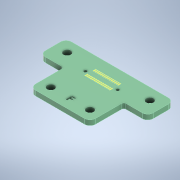
# Autodesk Inventor part: Out-facing Connector PCB
Saved by Autodesk Inventor 2021 (Build 250183000, 183)
## iProperties
Created: 2020-04-07
Part Number: Out-facing Connector PCB
Material: Phenolic Resin
Document SubType Name: Modeling
Designer: jgray
Density: 1.38 g/cm^3
Appearance: Smooth - Dark Sea Green
Author: jgray
Autodesk Inventor part; units mm, degrees
ref_plane "YZ Plane" through (0, 0, 0) normal (1, 0, 0) x (0, 1, 0)
ref_plane "XZ Plane" through (0, 0, 0) normal (0, 1, 0) x (-1, 0, 0)
ref_plane "XY Plane" through (0, 0, 0) normal (0, 0, 1) x (1, 0, 0)
sketch "Sketch1" plane through (0, 0, 0) normal (0, 1, 0) x (-1, 0, 0)
  line L0 (13.75, 0) -> (36.25, 0)
  line L1 (49.75, -18) -> (49.75, -25)
  line L2 (47.25, -27.5) -> (2.75, -27.5)
  line L3 (0.25, -25) -> (0.25, -18)
  line L4 (25, -34.1071) -> (25, 14.7902) construction
  line L5 (36.25, 0) -> (13.75, 0)
  line L6 (11.25, -2.5) -> (11.25, -14.5)
  line L7 (38.75, -14.5) -> (38.75, -2.5)
  line L8 (39.75, -15.5) -> (47.25, -15.5)
  line L9 (10.25, -15.5) -> (2.75, -15.5)
  arc A0 (38.75, -14.5) -> (39.75, -15.5) centre (39.75, -14.5) ccw
  arc A1 (10.25, -15.5) -> (11.25, -14.5) centre (10.25, -14.5) ccw
  arc A2 (49.75, -18) -> (47.25, -15.5) centre (47.25, -18) ccw
  arc A3 (47.25, -27.5) -> (49.75, -25) centre (47.25, -25) ccw
  arc A4 (2.75, -15.5) -> (0.25, -18) centre (2.75, -18) ccw
  arc A5 (0.25, -25) -> (2.75, -27.5) centre (2.75, -25) ccw
  arc A6 (38.75, -2.5) -> (36.25, 0) centre (36.25, -2.5) ccw
  arc A7 (13.75, 0) -> (11.25, -2.5) centre (13.75, -2.5) ccw
  point P0 (0, 0)
  point P1 (49.75, -27.5)
  point P2 (0.25, -27.5)
  point P3 (38.75, 0)
  point P4 (11.25, -1)
  point P5 (38.75, -1)
  point P6 (12.25, 0)
  dimension "d0" = 49.5
  dimension "d3" = 1
  dimension "d4" = 2.5
  dimension "d5" = 2.5
  dimension "d8" = 27.5
  dimension "d9" = 12
  dimension "d10" = 27.5
  dimension "d11" = 12
  dimension "d129" = 2.5
  dimension "d130" = 2.5
  constraints: 20 end point, 16 point on circle, 16 tangent, 10 point on line, 8 centre point, 3 equal radius, 3 parallel, 2 horizontal, 2 perpendicular, 1 vertical, 2 other
  measures "d0" distance of point (49.75, -27.5) point (0.25, -27.5)
  measures "d3" radius of A0
  measures "d4" radius of A2
  measures "d5" radius of A4
  measures "d8" distance between parallel lines of L2 L0
  measures "d9" distance between parallel lines of L2 L9
  measures "d10" distance between parallel lines of L7 L6
  measures "d11" distance between parallel lines of L2 L8
  measures "d129" radius of A6
  measures "d130" radius of A7
extrude "Extrusion1" add sketch "Sketch1" along normal blind 2.3
sketch "Sketch2" plane through (0, 2.3, 0) normal (0, 1, 0) x (1, 0, 0)
  line L0 (-48.4088, 22.25) -> (9.4819, 22.25) construction
  line L1 (-42.4458, 4.75) -> (-3.4379, 4.75) construction
  line L2 (-34, -3.7156) -> (-34, 9.7011) construction
  line L3 (-16, -3.7156) -> (-16, 9.7011) construction
  line L4 (-44, 10.4465) -> (-44, 20.1364) construction
  line L5 (-6, 8.2104) -> (-6, 20.1364) construction
  line L6 (-25, 27.2588) -> (-25, -6.0345) construction
  line L7 (-2.75, 27.5) -> (-47.25, 27.5) construction
  point P0 (0, 0)
  point P1 (-25, 27.5)
  point P2 (-44, 22.25)
  point P3 (-34, 4.75)
  point P4 (-16, 4.75)
  point P5 (-6, 22.25)
  dimension "d12" = 9
  dimension "d13" = 19
  dimension "d14" = 5.25
  dimension "d15" = 22.75
  constraints: 14 end point, 9 point on line, 4 vertical, 2 horizontal, 1 midpoint, 1 perpendicular, 2 other
  measures "d12" distance between parallel lines of L6 L3
  measures "d13" distance between parallel lines of L6 L4
  measures "d14" distance between parallel lines of L7 L0
  measures "d15" distance between parallel lines of L7 L1
hole "Hole1" at (-44, 2.3, -22.25) at (-34, 2.3, -4.75) at (-16, 2.3, -4.75) at (-6, 2.3, -22.25) direction (0, -1, 0) diameter 3.4 end through all clearance for "Countersunk Flat Head Screw ISO 2009/7046" size "M3" standard "ISO"
sketch "Sketch4" plane through (0, 2.3, 0) normal (0, 1, 0) x (1, 0, 0)
  circle A0 centre (-16, 4.75) radius 1.7 projected
  circle A1 centre (-44, 22.25) radius 1.7
  circle A2 centre (-34, 4.75) radius 1.7 projected
  circle A3 centre (-6, 22.25) radius 1.7 projected
  arc A4 (-10.25, 15.5) -> (-11.25, 14.5) centre (-10.25, 14.5) ccw projected
  line L0 (-10.25, 15.5) -> (-2.75, 15.5) projected
  arc A5 (-2.75, 15.5) -> (-0.25, 18) centre (-2.75, 18) ccw projected
  line L1 (-0.25, 18) -> (-0.25, 25) projected
  arc A6 (-0.25, 25) -> (-2.75, 27.5) centre (-2.75, 25) ccw projected
  line L2 (-2.75, 27.5) -> (-47.25, 27.5) projected
  arc A7 (-47.25, 27.5) -> (-49.75, 25) centre (-47.25, 25) ccw projected
  line L3 (-49.75, 25) -> (-49.75, 18) projected
  arc A8 (-49.75, 18) -> (-47.25, 15.5) centre (-47.25, 18) ccw projected
  line L4 (-47.25, 15.5) -> (-39.75, 15.5) projected
  arc A9 (-38.75, 14.5) -> (-39.75, 15.5) centre (-39.75, 14.5) ccw projected
  line L5 (-38.75, 14.5) -> (-38.75, 2.5) projected
  line L6 (-36.25, 0) -> (-13.75, 0) projected
  line L7 (-11.25, 2.5) -> (-11.25, 14.5) projected
  line L8 (-25, 29.284) -> (-25, -4.219) construction
  line L9 (-36.25, 0) -> (-13.75, 0) construction
  line L10 (-2.75, 27.5) -> (-47.25, 27.5) construction
  arc A10 (-13.75, 0) -> (-11.25, 2.5) centre (-13.75, 2.5) ccw projected
  arc A11 (-38.75, 2.5) -> (-36.25, 0) centre (-36.25, 2.5) ccw projected
  point P0 (0, 0)
  point P1 (-32.4, 19.05)
  point P2 (-17.6, 19.05)
  point P3 (-12.25, 0)
  point P4 (-25, 0)
  point P5 (-25, 27.5)
  point P6 (-25, 0)
  dimension "d29" = 14.8
  dimension "d45" = 7.4
  dimension "d47" = 14.3
  dimension "d48" = 14.3
  constraints: 3 midpoint, 3 point on line, 2 end point, 1 centre point
  measures "d29" distance of point (-17.6, 19.05) point (-32.4, 19.05)
  measures "d45" distance from line of point (-17.6, 19.05) L8
  measures "d47" vertical distance of A2.centre point (-17.6, 19.05)
  measures "d48" vertical distance of point (-32.4, 19.05) A2.centre
hole "Hole2" at (-32.4, 2.3, -19.05) at (-17.6, 2.3, -19.05) direction (0, -1, 0) diameter 1.45 end through all
sketch "Sketch3" plane through (0, 0, 0) normal (0, -1, 0) x (1, 0, 0)
  line L0 (-52.2125, -17.55) -> (3.151, -17.55) construction
  line L1 (-25, 3.9366) -> (-25, -33.6768) construction
  line L2 (-16, -20.35) -> (-34, -20.35)
  line L3 (-34, -20.35) -> (-34, -14.75)
  line L4 (-34, -14.75) -> (-16, -14.75)
  line L5 (-16, -14.75) -> (-16, -20.35)
  line L6 (-16, -20.35) -> (-34, -14.75) construction
  line L7 (-34, -20.35) -> (-16, -14.75) construction
  circle A0 centre (-16, -4.75) radius 1.7
  circle A1 centre (-34, -4.75) radius 1.7
  line L8 (-0.25, -15) -> (-0.25, -26.5)
  arc A2 (-1.25, -27.5) -> (-0.25, -26.5) centre (-1.25, -26.5) ccw
  line L9 (-1.25, -27.5) -> (-48.75, -27.5)
  arc A3 (-49.75, -26.5) -> (-48.75, -27.5) centre (-48.75, -26.5) ccw
  line L10 (-49.75, -26.5) -> (-49.75, -15)
  line L11 (-38.75, -13) -> (-38.75, -1)
  line L12 (-11.25, -1) -> (-11.25, -13)
  line L13 (-25.25, -19.25) -> (-25.25, -20.35)
  line L14 (-25.25, -20.35) -> (-24.75, -20.35)
  line L15 (-24.75, -20.35) -> (-24.75, -19.25)
  line L16 (-24.75, -19.25) -> (-25.25, -19.25)
  line L17 (-25.25, -19.25) -> (-24.75, -20.35) construction
  line L18 (-25.25, -20.35) -> (-24.75, -19.25) construction
  line L19 (-25.55, -20.35) -> (-25.55, -19.25)
  line L20 (-26.05, -19.25) -> (-26.05, -20.35)
  line L21 (-26.05, -20.35) -> (-25.55, -20.35)
  line L22 (-25.55, -19.25) -> (-26.05, -19.25)
  line L23 (-26.05, -20.35) -> (-25.55, -19.25) construction
  line L24 (-26.05, -19.25) -> (-25.55, -20.35) construction
  line L25 (-26.35, -20.35) -> (-26.35, -19.25)
  line L26 (-26.85, -19.25) -> (-26.85, -20.35)
  line L27 (-26.85, -20.35) -> (-26.35, -20.35)
  line L28 (-26.35, -19.25) -> (-26.85, -19.25)
  line L29 (-26.85, -20.35) -> (-26.35, -19.25) construction
  line L30 (-26.85, -19.25) -> (-26.35, -20.35) construction
  line L31 (-27.15, -20.35) -> (-27.15, -19.25)
  line L32 (-27.65, -19.25) -> (-27.65, -20.35)
  line L33 (-27.65, -20.35) -> (-27.15, -20.35)
  line L34 (-27.15, -19.25) -> (-27.65, -19.25)
  line L35 (-27.65, -20.35) -> (-27.15, -19.25) construction
  line L36 (-27.65, -19.25) -> (-27.15, -20.35) construction
  line L37 (-27.95, -20.35) -> (-27.95, -19.25)
  line L38 (-28.45, -19.25) -> (-28.45, -20.35)
  line L39 (-28.45, -20.35) -> (-27.95, -20.35)
  line L40 (-27.95, -19.25) -> (-28.45, -19.25)
  line L41 (-28.45, -20.35) -> (-27.95, -19.25) construction
  line L42 (-28.45, -19.25) -> (-27.95, -20.35) construction
  line L43 (-28.75, -20.35) -> (-28.75, -19.25)
  line L44 (-29.25, -19.25) -> (-29.25, -20.35)
  line L45 (-29.25, -20.35) -> (-28.75, -20.35)
  line L46 (-28.75, -19.25) -> (-29.25, -19.25)
  line L47 (-29.25, -20.35) -> (-28.75, -19.25) construction
  line L48 (-29.25, -19.25) -> (-28.75, -20.35) construction
  line L49 (-29.55, -20.35) -> (-29.55, -19.25)
  line L50 (-30.05, -19.25) -> (-30.05, -20.35)
  line L51 (-30.05, -20.35) -> (-29.55, -20.35)
  line L52 (-29.55, -19.25) -> (-30.05, -19.25)
  line L53 (-30.05, -20.35) -> (-29.55, -19.25) construction
  line L54 (-30.05, -19.25) -> (-29.55, -20.35) construction
  line L55 (-30.35, -20.35) -> (-30.35, -19.25)
  line L56 (-30.85, -19.25) -> (-30.85, -20.35)
  line L57 (-30.85, -20.35) -> (-30.35, -20.35)
  line L58 (-30.35, -19.25) -> (-30.85, -19.25)
  line L59 (-30.85, -20.35) -> (-30.35, -19.25) construction
  line L60 (-30.85, -19.25) -> (-30.35, -20.35) construction
  line L61 (-24.75, -15.85) -> (-24.75, -14.75)
  line L62 (-25.25, -14.75) -> (-25.25, -15.85)
  line L63 (-25.25, -15.85) -> (-24.75, -15.85)
  line L64 (-24.75, -14.75) -> (-25.25, -14.75)
  line L65 (-25.25, -15.85) -> (-24.75, -14.75) construction
  line L66 (-25.25, -14.75) -> (-24.75, -15.85) construction
  line L67 (-25.55, -15.85) -> (-25.55, -14.75)
  line L68 (-26.05, -14.75) -> (-26.05, -15.85)
  line L69 (-26.05, -15.85) -> (-25.55, -15.85)
  line L70 (-25.55, -14.75) -> (-26.05, -14.75)
  line L71 (-26.05, -15.85) -> (-25.55, -14.75) construction
  line L72 (-26.05, -14.75) -> (-25.55, -15.85) construction
  line L73 (-26.35, -15.85) -> (-26.35, -14.75)
  line L74 (-26.85, -14.75) -> (-26.85, -15.85)
  line L75 (-26.85, -15.85) -> (-26.35, -15.85)
  line L76 (-26.35, -14.75) -> (-26.85, -14.75)
  line L77 (-26.85, -15.85) -> (-26.35, -14.75) construction
  line L78 (-26.85, -14.75) -> (-26.35, -15.85) construction
  line L79 (-27.15, -15.85) -> (-27.15, -14.75)
  line L80 (-27.65, -14.75) -> (-27.65, -15.85)
  line L81 (-27.65, -15.85) -> (-27.15, -15.85)
  line L82 (-27.15, -14.75) -> (-27.65, -14.75)
  line L83 (-27.65, -15.85) -> (-27.15, -14.75) construction
  line L84 (-27.65, -14.75) -> (-27.15, -15.85) construction
  line L85 (-27.95, -15.85) -> (-27.95, -14.75)
  line L86 (-28.45, -14.75) -> (-28.45, -15.85)
  line L87 (-28.45, -15.85) -> (-27.95, -15.85)
  line L88 (-27.95, -14.75) -> (-28.45, -14.75)
  line L89 (-28.45, -15.85) -> (-27.95, -14.75) construction
  line L90 (-28.45, -14.75) -> (-27.95, -15.85) construction
  line L91 (-28.75, -15.85) -> (-28.75, -14.75)
  line L92 (-29.25, -14.75) -> (-29.25, -15.85)
  line L93 (-29.25, -15.85) -> (-28.75, -15.85)
  line L94 (-28.75, -14.75) -> (-29.25, -14.75)
  line L95 (-29.25, -15.85) -> (-28.75, -14.75) construction
  line L96 (-29.25, -14.75) -> (-28.75, -15.85) construction
  line L97 (-29.55, -15.85) -> (-29.55, -14.75)
  line L98 (-30.05, -14.75) -> (-30.05, -15.85)
  line L99 (-30.05, -15.85) -> (-29.55, -15.85)
  line L100 (-29.55, -14.75) -> (-30.05, -14.75)
  line L101 (-30.05, -15.85) -> (-29.55, -14.75) construction
  line L102 (-30.05, -14.75) -> (-29.55, -15.85) construction
  line L103 (-30.35, -15.85) -> (-30.35, -14.75)
  line L104 (-30.85, -14.75) -> (-30.85, -15.85)
  line L105 (-30.85, -15.85) -> (-30.35, -15.85)
  line L106 (-30.35, -14.75) -> (-30.85, -14.75)
  line L107 (-30.85, -15.85) -> (-30.35, -14.75) construction
  line L108 (-30.85, -14.75) -> (-30.35, -15.85) construction
  line L109 (-23.95, -20.35) -> (-23.95, -19.25)
  line L110 (-24.45, -19.25) -> (-24.45, -20.35)
  line L111 (-24.45, -20.35) -> (-23.95, -20.35)
  line L112 (-23.95, -19.25) -> (-24.45, -19.25)
  line L113 (-24.45, -19.25) -> (-23.95, -20.35) construction
  line L114 (-24.45, -20.35) -> (-23.95, -19.25) construction
  line L115 (-23.15, -20.35) -> (-23.15, -19.25)
  line L116 (-23.65, -19.25) -> (-23.65, -20.35)
  line L117 (-23.65, -20.35) -> (-23.15, -20.35)
  line L118 (-23.15, -19.25) -> (-23.65, -19.25)
  line L119 (-23.65, -19.25) -> (-23.15, -20.35) construction
  line L120 (-23.65, -20.35) -> (-23.15, -19.25) construction
  line L121 (-22.35, -20.35) -> (-22.35, -19.25)
  line L122 (-22.85, -19.25) -> (-22.85, -20.35)
  line L123 (-22.85, -20.35) -> (-22.35, -20.35)
  line L124 (-22.35, -19.25) -> (-22.85, -19.25)
  line L125 (-22.85, -19.25) -> (-22.35, -20.35) construction
  line L126 (-22.85, -20.35) -> (-22.35, -19.25) construction
  line L127 (-21.55, -20.35) -> (-21.55, -19.25)
  line L128 (-22.05, -19.25) -> (-22.05, -20.35)
  line L129 (-22.05, -20.35) -> (-21.55, -20.35)
  line L130 (-21.55, -19.25) -> (-22.05, -19.25)
  line L131 (-22.05, -19.25) -> (-21.55, -20.35) construction
  line L132 (-22.05, -20.35) -> (-21.55, -19.25) construction
  line L133 (-20.75, -20.35) -> (-20.75, -19.25)
  line L134 (-21.25, -19.25) -> (-21.25, -20.35)
  line L135 (-21.25, -20.35) -> (-20.75, -20.35)
  line L136 (-20.75, -19.25) -> (-21.25, -19.25)
  line L137 (-21.25, -19.25) -> (-20.75, -20.35) construction
  line L138 (-21.25, -20.35) -> (-20.75, -19.25) construction
  line L139 (-19.95, -20.35) -> (-19.95, -19.25)
  line L140 (-20.45, -19.25) -> (-20.45, -20.35)
  line L141 (-20.45, -20.35) -> (-19.95, -20.35)
  line L142 (-19.95, -19.25) -> (-20.45, -19.25)
  line L143 (-20.45, -19.25) -> (-19.95, -20.35) construction
  line L144 (-20.45, -20.35) -> (-19.95, -19.25) construction
  line L145 (-19.15, -20.35) -> (-19.15, -19.25)
  line L146 (-19.65, -19.25) -> (-19.65, -20.35)
  line L147 (-19.65, -20.35) -> (-19.15, -20.35)
  line L148 (-19.15, -19.25) -> (-19.65, -19.25)
  line L149 (-19.65, -19.25) -> (-19.15, -20.35) construction
  line L150 (-19.65, -20.35) -> (-19.15, -19.25) construction
  line L151 (-24.75, -15.85) -> (-24.75, -14.75)
  line L152 (-25.25, -14.75) -> (-25.25, -15.85)
  line L153 (-25.25, -15.85) -> (-24.75, -15.85)
  line L154 (-24.75, -14.75) -> (-25.25, -14.75)
  line L155 (-25.25, -14.75) -> (-24.75, -15.85) construction
  line L156 (-25.25, -15.85) -> (-24.75, -14.75) construction
  line L157 (-23.95, -15.85) -> (-23.95, -14.75)
  line L158 (-24.45, -14.75) -> (-24.45, -15.85)
  line L159 (-24.45, -15.85) -> (-23.95, -15.85)
  line L160 (-23.95, -14.75) -> (-24.45, -14.75)
  line L161 (-24.45, -14.75) -> (-23.95, -15.85) construction
  line L162 (-24.45, -15.85) -> (-23.95, -14.75) construction
  line L163 (-23.15, -15.85) -> (-23.15, -14.75)
  line L164 (-23.65, -14.75) -> (-23.65, -15.85)
  line L165 (-23.65, -15.85) -> (-23.15, -15.85)
  line L166 (-23.15, -14.75) -> (-23.65, -14.75)
  line L167 (-23.65, -14.75) -> (-23.15, -15.85) construction
  line L168 (-23.65, -15.85) -> (-23.15, -14.75) construction
  line L169 (-22.35, -15.85) -> (-22.35, -14.75)
  line L170 (-22.85, -14.75) -> (-22.85, -15.85)
  line L171 (-22.85, -15.85) -> (-22.35, -15.85)
  line L172 (-22.35, -14.75) -> (-22.85, -14.75)
  line L173 (-22.85, -14.75) -> (-22.35, -15.85) construction
  line L174 (-22.85, -15.85) -> (-22.35, -14.75) construction
  line L175 (-21.55, -15.85) -> (-21.55, -14.75)
  line L176 (-22.05, -14.75) -> (-22.05, -15.85)
  line L177 (-22.05, -15.85) -> (-21.55, -15.85)
  line L178 (-21.55, -14.75) -> (-22.05, -14.75)
  line L179 (-22.05, -14.75) -> (-21.55, -15.85) construction
  line L180 (-22.05, -15.85) -> (-21.55, -14.75) construction
  line L181 (-20.75, -15.85) -> (-20.75, -14.75)
  line L182 (-21.25, -14.75) -> (-21.25, -15.85)
  line L183 (-21.25, -15.85) -> (-20.75, -15.85)
  line L184 (-20.75, -14.75) -> (-21.25, -14.75)
  line L185 (-21.25, -14.75) -> (-20.75, -15.85) construction
  line L186 (-21.25, -15.85) -> (-20.75, -14.75) construction
  line L187 (-19.95, -15.85) -> (-19.95, -14.75)
  line L188 (-20.45, -14.75) -> (-20.45, -15.85)
  line L189 (-20.45, -15.85) -> (-19.95, -15.85)
  line L190 (-19.95, -14.75) -> (-20.45, -14.75)
  line L191 (-20.45, -14.75) -> (-19.95, -15.85) construction
  line L192 (-20.45, -15.85) -> (-19.95, -14.75) construction
  line L193 (-19.15, -15.85) -> (-19.15, -14.75)
  line L194 (-19.65, -14.75) -> (-19.65, -15.85)
  line L195 (-19.65, -15.85) -> (-19.15, -15.85)
  line L196 (-19.15, -14.75) -> (-19.65, -14.75)
  line L197 (-19.65, -14.75) -> (-19.15, -15.85) construction
  line L198 (-19.65, -15.85) -> (-19.15, -14.75) construction
  point P0 (-25, -17.55)
  point P1 (-25, -3.9366)
  point P2 (-32.4, -19.05)
  point P3 (-17.6, -19.05)
  point P4 (-25, -19.8)
  point P5 (-25.8, -19.8)
  point P6 (-26.6, -19.8)
  point P7 (-27.4, -19.8)
  point P8 (-28.2, -19.8)
  point P9 (-29, -19.8)
  point P10 (-29.8, -19.8)
  point P11 (-30.6, -19.8)
  point P12 (-25, -15.3)
  point P13 (-25.8, -15.3)
  point P14 (-26.6, -15.3)
  point P15 (-27.4, -15.3)
  point P16 (-28.2, -15.3)
  point P17 (-29, -15.3)
  point P18 (-29.8, -15.3)
  point P19 (-30.6, -15.3)
  point P20 (-24.2, -19.8)
  point P21 (-23.4, -19.8)
  point P22 (-22.6, -19.8)
  point P23 (-21.8, -19.8)
  point P24 (-21, -19.8)
  point P25 (-20.2, -19.8)
  point P26 (-19.4, -19.8)
  point P27 (-25, -15.3)
  point P28 (-24.2, -15.3)
  point P29 (-23.4, -15.3)
  point P30 (-22.6, -15.3)
  point P31 (-21.8, -15.3)
  point P32 (-21, -15.3)
  point P33 (-20.2, -15.3)
  point P34 (-19.4, -15.3)
  dimension "d24" = 18
  dimension "d25" = 5.6
  dimension "d41" = 1.5
  dimension "d42" = 2.8
  dimension "d104" = 0.5
  dimension "d106" = 14.8
  dimension "d107" = 7.15
  dimension "d108" = 1.1
  dimension "d109" = 1.1
  dimension "d112" = 0.8
  dimension "d115" = 4.5
  dimension "d120" = 0.8
  dimension "d123" = 4.5
  dimension "d133" = 7.4
  dimension "d134" = 1.5
  constraints: 394 end point, 70 horizontal alignment, 64 midpoint, 59 parallel, 28 collinear, 4 centre point, 4 point on circle, 4 vertical, 3 point on line, 1 horizontal, 1 perpendicular, 182 other
  measures "d24" distance of L3.end L5.start
  measures "d25" distance of L3.start L3.end
  measures "d41" distance from line of point (-17.6, -19.05) L0
  measures "d104" distance of L14.end L13.end
  measures "d106" distance of point (-32.4, -19.05) point (-17.6, -19.05)
  measures "d109" distance between parallel lines of L14 L16
  measures "d112" distance of L15.end L19.end
  measures "d115" distance of L15.end L61.end
  measures "d120" distance of L14.end L109.start
  measures "d123" distance of L14.end L151.start
  measures "d133" distance from line of point (-32.4, -19.05) L1
  measures "d134" distance from line of point (-32.4, -19.05) L0
sketch "Sketch5" plane through (0, 2.3, 0) normal (0, 1, 0) x (1, 0, 0)
  line L0 (-52.8164, 19.64) -> (4.9571, 19.64) construction
  line L1 (-2.75, 27.5) -> (-47.25, 27.5) construction
  line L2 (-25, 27.5) -> (-25, -1.2167) construction
  line L3 (-25.275, 22.29) -> (-25.275, 20.79)
  line L4 (-25.275, 20.79) -> (-24.725, 20.79)
  line L5 (-24.725, 20.79) -> (-24.725, 22.29)
  line L6 (-24.725, 22.29) -> (-25.275, 22.29)
  line L7 (-25.275, 22.29) -> (-23.775, 22.29) construction
  line L8 (-24.475, 22.29) -> (-24.475, 20.79)
  line L9 (-24.475, 20.79) -> (-23.925, 20.79)
  line L10 (-23.925, 20.79) -> (-23.925, 22.29)
  line L11 (-23.925, 22.29) -> (-24.475, 22.29)
  line L12 (-23.675, 22.29) -> (-23.675, 20.79)
  line L13 (-23.675, 20.79) -> (-23.125, 20.79)
  line L14 (-23.125, 20.79) -> (-23.125, 22.29)
  line L15 (-23.125, 22.29) -> (-23.675, 22.29)
  line L16 (-22.875, 22.29) -> (-22.875, 20.79)
  line L17 (-22.875, 20.79) -> (-22.325, 20.79)
  line L18 (-22.325, 20.79) -> (-22.325, 22.29)
  line L19 (-22.325, 22.29) -> (-22.875, 22.29)
  line L20 (-22.075, 22.29) -> (-22.075, 20.79)
  line L21 (-22.075, 20.79) -> (-21.525, 20.79)
  line L22 (-21.525, 20.79) -> (-21.525, 22.29)
  line L23 (-21.525, 22.29) -> (-22.075, 22.29)
  line L24 (-21.275, 22.29) -> (-21.275, 20.79)
  line L25 (-21.275, 20.79) -> (-20.725, 20.79)
  line L26 (-20.725, 20.79) -> (-20.725, 22.29)
  line L27 (-20.725, 22.29) -> (-21.275, 22.29)
  line L28 (-20.475, 22.29) -> (-20.475, 20.79)
  line L29 (-20.475, 20.79) -> (-19.925, 20.79)
  line L30 (-19.925, 20.79) -> (-19.925, 22.29)
  line L31 (-19.925, 22.29) -> (-20.475, 22.29)
  line L32 (-25.525, 20.79) -> (-25.525, 22.29)
  line L33 (-26.075, 20.79) -> (-25.525, 20.79)
  line L34 (-25.525, 22.29) -> (-26.075, 22.29)
  line L35 (-26.075, 22.29) -> (-26.075, 20.79)
  line L36 (-26.325, 20.79) -> (-26.325, 22.29)
  line L37 (-26.875, 20.79) -> (-26.325, 20.79)
  line L38 (-26.325, 22.29) -> (-26.875, 22.29)
  line L39 (-26.875, 22.29) -> (-26.875, 20.79)
  line L40 (-27.125, 20.79) -> (-27.125, 22.29)
  line L41 (-27.675, 20.79) -> (-27.125, 20.79)
  line L42 (-27.125, 22.29) -> (-27.675, 22.29)
  line L43 (-27.675, 22.29) -> (-27.675, 20.79)
  line L44 (-27.925, 20.79) -> (-27.925, 22.29)
  line L45 (-28.475, 20.79) -> (-27.925, 20.79)
  line L46 (-27.925, 22.29) -> (-28.475, 22.29)
  line L47 (-28.475, 22.29) -> (-28.475, 20.79)
  line L48 (-28.725, 20.79) -> (-28.725, 22.29)
  line L49 (-29.275, 20.79) -> (-28.725, 20.79)
  line L50 (-28.725, 22.29) -> (-29.275, 22.29)
  line L51 (-29.275, 22.29) -> (-29.275, 20.79)
  line L52 (-29.525, 20.79) -> (-29.525, 22.29)
  line L53 (-30.075, 20.79) -> (-29.525, 20.79)
  line L54 (-29.525, 22.29) -> (-30.075, 22.29)
  line L55 (-30.075, 22.29) -> (-30.075, 20.79)
  line L56 (-25.275, 16.99) -> (-24.725, 16.99)
  line L57 (-24.725, 18.49) -> (-25.275, 18.49)
  line L58 (-25.275, 18.49) -> (-25.275, 16.99)
  line L59 (-25.275, 18.49) -> (-23.775, 18.49) construction
  line L60 (-23.125, 16.99) -> (-23.125, 18.49)
  line L61 (-23.675, 16.99) -> (-23.125, 16.99)
  line L62 (-23.125, 18.49) -> (-23.675, 18.49)
  line L63 (-22.875, 18.49) -> (-22.875, 16.99)
  line L64 (-22.325, 18.49) -> (-22.875, 18.49)
  line L65 (-22.875, 16.99) -> (-22.325, 16.99)
  line L66 (-22.325, 16.99) -> (-22.325, 18.49)
  line L67 (-22.075, 18.49) -> (-22.075, 16.99)
  line L68 (-21.525, 18.49) -> (-22.075, 18.49)
  line L69 (-22.075, 16.99) -> (-21.525, 16.99)
  line L70 (-21.525, 16.99) -> (-21.525, 18.49)
  line L71 (-21.275, 18.49) -> (-21.275, 16.99)
  line L72 (-20.725, 18.49) -> (-21.275, 18.49)
  line L73 (-21.275, 16.99) -> (-20.725, 16.99)
  line L74 (-20.725, 16.99) -> (-20.725, 18.49)
  line L75 (-20.475, 18.49) -> (-20.475, 16.99)
  line L76 (-20.475, 16.99) -> (-19.925, 16.99)
  line L77 (-19.925, 16.99) -> (-19.925, 18.49)
  line L78 (-19.925, 18.49) -> (-20.475, 18.49)
  line L79 (-25.525, 16.99) -> (-25.525, 18.49)
  line L80 (-25.525, 18.49) -> (-26.075, 18.49)
  line L81 (-26.075, 16.99) -> (-25.525, 16.99)
  line L82 (-26.075, 18.49) -> (-26.075, 16.99)
  line L83 (-26.325, 16.99) -> (-26.325, 18.49)
  line L84 (-26.875, 18.49) -> (-26.875, 16.99)
  line L85 (-26.325, 18.49) -> (-26.875, 18.49)
  line L86 (-26.875, 16.99) -> (-26.325, 16.99)
  line L87 (-27.675, 16.99) -> (-27.125, 16.99)
  line L88 (-27.675, 18.49) -> (-27.675, 16.99)
  line L89 (-27.125, 18.49) -> (-27.675, 18.49)
  line L90 (-27.925, 16.99) -> (-27.925, 18.49)
  line L91 (-28.475, 16.99) -> (-27.925, 16.99)
  line L92 (-28.475, 18.49) -> (-28.475, 16.99)
  line L93 (-27.925, 18.49) -> (-28.475, 18.49)
  line L94 (-27.125, 16.99) -> (-27.125, 18.49)
  line L95 (-28.725, 16.99) -> (-28.725, 18.49)
  line L96 (-29.275, 16.99) -> (-28.725, 16.99)
  line L97 (-28.725, 18.49) -> (-29.275, 18.49)
  line L98 (-29.275, 18.49) -> (-29.275, 16.99)
  line L99 (-29.525, 16.99) -> (-29.525, 18.49)
  line L100 (-30.075, 16.99) -> (-29.525, 16.99)
  line L101 (-30.075, 18.49) -> (-30.075, 16.99)
  line L102 (-29.525, 18.49) -> (-30.075, 18.49)
  line L103 (-24.475, 16.99) -> (-23.925, 16.99)
  line L104 (-24.725, 16.99) -> (-24.725, 18.49)
  line L105 (-24.475, 18.49) -> (-24.475, 16.99)
  line L106 (-23.925, 18.49) -> (-24.475, 18.49)
  line L107 (-23.925, 16.99) -> (-23.925, 18.49)
  line L108 (-23.675, 18.49) -> (-23.675, 16.99)
  line L109 (-19.675, 22.29) -> (-19.675, 20.79)
  line L110 (-19.675, 20.79) -> (-19.125, 20.79)
  line L111 (-19.125, 20.79) -> (-19.125, 22.29)
  line L112 (-19.125, 22.29) -> (-19.675, 22.29)
  line L113 (-19.675, 18.49) -> (-19.675, 16.99)
  line L114 (-19.675, 16.99) -> (-19.125, 16.99)
  line L115 (-19.125, 16.99) -> (-19.125, 18.49)
  line L116 (-19.125, 18.49) -> (-19.675, 18.49)
  line L117 (-30.325, 20.79) -> (-30.325, 22.29)
  line L118 (-30.875, 20.79) -> (-30.325, 20.79)
  line L119 (-30.325, 22.29) -> (-30.875, 22.29)
  line L120 (-30.875, 22.29) -> (-30.875, 20.79)
  line L121 (-30.325, 16.99) -> (-30.325, 18.49)
  line L122 (-30.875, 16.99) -> (-30.325, 16.99)
  line L123 (-30.875, 18.49) -> (-30.875, 16.99)
  line L124 (-30.325, 18.49) -> (-30.875, 18.49)
  point P0 (0, 0)
  point P1 (-25, 21.6605)
  point P2 (-24.2, 21.6605)
  point P3 (-23.4, 21.6605)
  point P4 (-22.6, 21.6605)
  point P5 (-21.8, 21.6605)
  point P6 (-21, 21.6605)
  point P7 (-20.2, 21.6605)
  point P8 (-25.8, 21.6605)
  point P9 (-26.6, 21.6605)
  point P10 (-27.4, 21.6605)
  point P11 (-28.2, 21.6605)
  point P12 (-29, 21.6605)
  point P13 (-29.8, 21.6605)
  point P14 (-23.4, 17.8605)
  point P15 (-22.6, 17.8605)
  point P16 (-21.8, 17.8605)
  point P17 (-20.2, 17.8605)
  point P18 (-21, 17.8605)
  point P19 (-25.8, 17.8605)
  point P20 (-26.6, 17.8605)
  point P21 (-27.4, 17.8605)
  point P22 (-28.2, 17.8605)
  point P23 (-29, 17.8605)
  point P24 (-29.8, 17.8605)
  point P25 (-25, 17.8605)
  point P26 (-24.2, 17.8605)
  point P27 (-19.4, 21.6605)
  point P28 (-19.4, 17.8605)
  point P29 (-30.6, 21.6605)
  point P30 (-30.6, 17.8605)
  dimension "d49" = 7.86
  dimension "d50" = 1.5
  dimension "d51" = 90
  dimension "d52" = 0.55
  dimension "d55" = 0.8
  dimension "d62" = 0.8
  dimension "d69" = 3.8
  dimension "d74" = 1.15
  dimension "d75" = 1.15
  dimension "d102" = 0.8
  dimension "d103" = 0.8
  constraints: 248 end point, 4 horizontal, 3 parallel, 2 midpoint, 2 perpendicular, 2 point on line, 2 vertical, 227 other
  measures "d49" distance between parallel lines of L1 L0
  measures "d50" distance of L3.start L3.end
  measures "d51" angle of L3 L7
  measures "d52" distance of L4.end L3.end
  measures "d55" distance of L3.start L8.start
  measures "d62" distance of L4.end L32.start
  measures "d69" distance of L3.end L56.start
  measures "d74" distance between parallel lines of L102 L0
  measures "d75" distance between parallel lines of L45 L0
  measures "d102" distance of point (-29.8, 21.661) point (-30.6, 21.661)
  measures "d103" distance of point (-20.2, 21.661) point (-19.4, 21.661)
extrude "Extrusion2" add sketch "Sketch5" along normal blind 0.01
extrude "Extrusion3" add sketch "Sketch3" along normal blind 0.005 contours L2 L146 L148 L145 | L193 L195 L194 L4 | L2 L140 L142 L139 | L187 L189 L188 L4 | L2 L134 L136 L133 | L181 L183 L182 L4 | L2 L128 L130 L127 | L175 L177 L176 L4 | L2 L122 L124 L121 | L169 L171 L170 L4 | L2 L116 L118 L115 | L163 L165 L164 L4 | L2 L110 L112 L109 | L157 L159 L158 L4 | L2 L13 L16 L15 | L61 L63 L62 L4 | L2 L20 L22 L19 | L67 L69 L68 L4 | L2 L26 L28 L25 | L73 L75 L74 L4 | L2 L32 L34 L31 | L79 L81 L80 L4 | L2 L38 L40 L37 | L85 L87 L86 L4 | L2 L44 L46 L43 | L91 L93 L92 L4 | L2 L50 L52 L49 | L97 L99 L98 L4 | L2 L56 L58 L55 | L103 L105 L104 L4
sketch "Sketch6" plane through (0, 2.3, 0) normal (0, 1, 0) x (1, 0, 0)
  line L0 (-26.0842, 6.1798) -> (-20.3705, 6.1798) construction
  line L1 (-20.3705, 6.1798) -> (-20.3705, 2.1201) construction
  line L2 (-20.3705, 2.1201) -> (-26.0842, 2.1201) construction
  line L3 (-26.0842, 2.1201) -> (-26.0842, 6.1798) construction
  line L4 (-23.7649, 5.6085) -> (-25.0243, 5.6085)
  line L5 (-25.0243, 5.6085) -> (-25.0243, 5.042)
  line L6 (-25.0243, 5.042) -> (-23.8646, 5.042)
  line L7 (-23.8646, 5.042) -> (-23.8646, 4.4707)
  line L8 (-23.8646, 4.4707) -> (-25.0243, 4.4707)
  line L9 (-25.0243, 4.4707) -> (-25.0243, 3.1798)
  line L10 (-25.0243, 3.1798) -> (-25.7731, 3.1798)
  line L11 (-25.7731, 3.1798) -> (-25.7731, 6.1798)
  line L12 (-25.7731, 6.1798) -> (-23.7649, 6.1798)
  line L13 (-23.7649, 6.1798) -> (-23.7649, 5.6085)
  point P0 (0, 0)
  constraints: 2 other
emboss "Emboss1" sketch "Sketch6" operation cut depth 2.6 direction (0, -1, 0)
equation "\"d11\" = d9"
body "Solid1"
